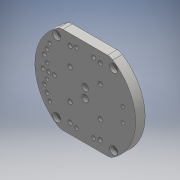
# Autodesk Inventor part: Modular Chassis
Saved by Autodesk Inventor 2016 (Build 200138000, 138)
## iProperties
Created: 2017-03-04
Part Number: Modular Chassis
Material: Generic
Document SubType Name: Modeling
Designer: Billy
Density: 1 g/cm^3
Appearance: Default
Author: Billy
Autodesk Inventor part; units mm, degrees
ref_plane "YZ Plane" through (0, 0, 0) normal (1, 0, 0) x (0, 1, 0)
ref_plane "XZ Plane" through (0, 0, 0) normal (0, 1, 0) x (-1, 0, 0)
ref_plane "XY Plane" through (0, 0, 0) normal (0, 0, 1) x (1, 0, 0)
sketch "Sketch1" plane through (0, 0, 0) normal (0, 1, 0) x (-1, 0, 0)
  circle A0 centre (15.9, 35) radius 2.25
  circle A1 centre (-15.9, 35) radius 2.25
  circle A2 centre (15.9, 16) radius 2.25
  circle A3 centre (-15.9, 16) radius 2.25
  circle A4 centre (0, 0) radius 50.311529
  circle A5 centre (15.9, -35) radius 2.25
  circle A6 centre (-15.9, -35) radius 2.25
  circle A7 centre (15.9, -16) radius 2.25
  circle A8 centre (-15.9, -16) radius 2.25
  circle A9 centre (9, 36.699372) radius 2
  circle A10 centre (-9, 36.699372) radius 2
  circle A11 centre (9, -36.699372) radius 2
  circle A12 centre (-9, -36.699372) radius 2
  circle A13 centre (39.811529, 7.366) radius 1.75
  circle A14 centre (39.811529, -7.366) radius 1.75
  circle A15 centre (-39.811529, 7.366) radius 1.75
  circle A16 centre (-39.811529, -7.366) radius 1.75
  circle A17 centre (27.855765, 21.183) radius 1.5
  circle A18 centre (30.740586, 14.805085) radius 1.5
  circle A19 centre (24.970943, 27.560915) radius 1.5
  circle A20 centre (27.855765, -21.183) radius 1.5
  circle A21 centre (30.740586, -14.805085) radius 1.5
  circle A22 centre (24.970943, -27.560915) radius 1.5
  circle A23 centre (0, 32.311529) radius 2
  circle A24 centre (0, 38.311529) radius 2
  circle A25 centre (0, 44.311529) radius 2
  circle A26 centre (-32.311529, 0) radius 2
  circle A27 centre (-38.311529, 0) radius 2
  circle A28 centre (-44.311529, 0) radius 2
  circle A29 centre (0, -32.311529) radius 2
  circle A30 centre (0, -38.311529) radius 2
  circle A31 centre (0, -44.311529) radius 2
  circle A32 centre (32.311529, 0) radius 2
  circle A33 centre (38.311529, 0) radius 2
  circle A34 centre (44.311529, 0) radius 2
  circle A35 centre (0, 5) radius 2.5
  circle A36 centre (0, -5) radius 2.5
  circle A37 centre (24.105765, 8) radius 2
  circle A38 centre (24.105765, -8) radius 2
  circle A39 centre (-24.105765, 8) radius 2
  circle A40 centre (-24.105765, -8) radius 2
  circle A41 centre (-27.855765, -21.183) radius 2
  circle A42 centre (27.885979, -37.390623) radius 2
  line L0 (0, 0) -> (2.5, 0)
  circle A43 centre (27.885979, 37.390623) radius 2
  circle A44 centre (44.311529, -14.732) radius 2
  circle A45 centre (44.311529, 14.732) radius 2
  line L1 (-27.855765, -21.183) -> (-36.920676, -29.026812)
  circle A46 centre (-21.877882, -28.0915) radius 2
  circle A47 centre (-33.833647, -14.2745) radius 2
  circle A48 centre (-27.927504, -33.3262) radius 2
  circle A49 centre (-33.905386, -26.4177) radius 2
  circle A50 centre (-39.883268, -19.5092) radius 2
  circle A51 centre (-27.855765, 21.183) radius 2
  circle A52 centre (-21.877882, 28.0915) radius 2
  circle A53 centre (-33.833647, 14.2745) radius 2
  circle A54 centre (-27.927504, 33.3262) radius 2
  circle A55 centre (-33.905386, 26.4177) radius 2
  circle A56 centre (-39.883268, 19.5092) radius 2
  circle A57 centre (36.098754, -26.061311) radius 2
  circle A58 centre (36.098754, 26.061311) radius 2
  point P0 (-36.920676, 29.026812)
  dimension "d47" = 360
  dimension "d64" = 8
  dimension "d69" = 4
  dimension "d70" = 4
  constraints: 59 centre point, 9 symmetric about line, 4 end point, 1 horizontal, 40 other
  measures "d64" distance of A46.centre A48.centre
  measures "d69" diameter of A57
  measures "d70" diameter of A58
extrude "Extrusion1" add sketch "Sketch1" along normal blind 10
sketch "Sketch2" plane through (0, 10, 0) normal (0, 1, 0) x (1, 0, 0)
  circle A0 centre (0, 5) radius 2.5
  circle A1 centre (0, -5) radius 2.5
  circle A2 centre (15.9, 16) radius 2.25
  circle A3 centre (-15.9, 16) radius 2.25
  circle A4 centre (15.9, 35) radius 2.25
  circle A5 centre (-15.9, 35) radius 2.25
  circle A6 centre (15.9, -16) radius 2.25
  circle A7 centre (-15.9, -16) radius 2.25
  circle A8 centre (15.9, -35) radius 2.25
  circle A9 centre (-36.098754, -26.061311) radius 2
  circle A10 centre (-36.098754, 26.061311) radius 2
  circle A11 centre (27.927504, -33.3262) radius 2
  circle A12 centre (39.883268, -19.5092) radius 2
  circle A13 centre (33.833647, -14.2745) radius 2
  circle A14 centre (27.855765, -21.183) radius 2
  circle A15 centre (33.905386, -26.4177) radius 2
  circle A16 centre (21.877882, -28.0915) radius 2
  circle A17 centre (39.883268, 19.5092) radius 2
  circle A18 centre (33.905386, 26.4177) radius 2
  circle A19 centre (27.927504, 33.3262) radius 2
  circle A20 centre (33.833647, 14.2745) radius 2
  circle A21 centre (21.877882, 28.0915) radius 2
  circle A22 centre (-44.311529, -14.732) radius 2
  circle A23 centre (-44.311529, 14.732) radius 2
  circle A24 centre (-27.885979, -37.390623) radius 2
  circle A25 centre (-27.885979, 37.390623) radius 2
  circle A26 centre (27.855765, 21.183) radius 2
  circle A27 centre (24.105765, 8) radius 2
  circle A28 centre (24.105765, -8) radius 2
  circle A29 centre (-24.105765, 8) radius 2
  circle A30 centre (-24.105765, -8) radius 2
  circle A31 centre (-44.311529, 0) radius 2
  circle A32 centre (-38.311529, 0) radius 2
  circle A33 centre (-32.311529, 0) radius 2
  circle A34 centre (0, 44.311529) radius 2
  circle A35 centre (0, 38.311529) radius 2
  circle A36 centre (0, 32.311529) radius 2
  circle A37 centre (44.311529, 0) radius 2
  circle A38 centre (38.311529, 0) radius 2
  circle A39 centre (32.311529, 0) radius 2
  circle A40 centre (0, -44.311529) radius 2
  circle A41 centre (0, -38.311529) radius 2
  circle A42 centre (0, -32.311529) radius 2
  circle A43 centre (-9, 36.699372) radius 2
  circle A44 centre (9, 36.699372) radius 2
  circle A45 centre (9, -36.699372) radius 2
  circle A46 centre (39.811529, 7.366) radius 1.75
  circle A47 centre (39.811529, -7.366) radius 1.75
  circle A48 centre (-39.811529, 7.366) radius 1.75
  circle A49 centre (-39.811529, -7.366) radius 1.75
  circle A50 centre (-30.740586, 14.805085) radius 1.5
  circle A51 centre (-27.855765, 21.183) radius 1.5
  circle A52 centre (-24.970943, 27.560915) radius 1.5
  circle A53 centre (-24.970943, -27.560915) radius 1.5
  circle A54 centre (-30.740586, -14.805085) radius 1.5
  circle A55 centre (-27.855765, -21.183) radius 1.5
  circle A56 centre (0, 0) radius 50.311529
  circle A57 centre (44.311529, 0) radius 2
  circle A58 centre (38.311529, 0) radius 2
  circle A59 centre (32.311529, 0) radius 2
  circle A60 centre (39.811529, 7.366) radius 1.75
  circle A61 centre (39.811529, -7.366) radius 1.75
  circle A62 centre (-15.9, -16) radius 5
  arc A63 (-14.704301, -30.145074) -> (-17.095699, -39.854926) centre (-15.9, -35) ccw
  arc A64 (-10.195699, -41.554298) -> (-7.804301, -31.844446) centre (-9, -36.699372) ccw
  line L0 (-10.195699, -41.554298) -> (-17.095699, -39.854926)
  circle A65 centre (-15.9, -35) radius 2.25
  circle A66 centre (-9, -36.699372) radius 2
  line L1 (-7.804301, -31.844446) -> (-14.704301, -30.145074)
  line L2 (0, 0) -> (0, -5)
  line L3 (0, 0) -> (-3.620732, 0)
  circle A67 centre (15.9, -16) radius 5
  arc A68 (17.095699, -39.854926) -> (14.704301, -30.145074) centre (15.9, -35) ccw
  arc A69 (7.804301, -31.844446) -> (10.195699, -41.554298) centre (9, -36.699372) ccw
  line L4 (10.195699, -41.554298) -> (17.095699, -39.854926)
  line L5 (7.804301, -31.844446) -> (14.704301, -30.145074)
  circle A70 centre (-15.9, 16) radius 5
  arc A71 (-17.095699, 39.854926) -> (-14.704301, 30.145074) centre (-15.9, 35) ccw
  arc A72 (-7.804301, 31.844446) -> (-10.195699, 41.554298) centre (-9, 36.699372) ccw
  line L6 (-10.195699, 41.554298) -> (-17.095699, 39.854926)
  line L7 (-7.804301, 31.844446) -> (-14.704301, 30.145074)
  arc A73 (14.704301, 30.145074) -> (17.095699, 39.854926) centre (15.9, 35) ccw
  line L8 (7.804301, 31.844446) -> (14.704301, 30.145074)
  arc A74 (10.195699, 41.554298) -> (7.804301, 31.844446) centre (9, 36.699372) ccw
  line L9 (10.195699, 41.554298) -> (17.095699, 39.854926)
  circle A75 centre (15.9, 16) radius 5
  circle A76 centre (-39.811529, 7.366) radius 4.25
  circle A77 centre (-39.811529, -7.366) radius 4.25
  circle A78 centre (39.811529, 7.366) radius 4.25
  circle A79 centre (39.811529, -7.366) radius 4.25
  dimension "d85" = 8.5
  dimension "d86" = 8.5
  dimension "d87" = 8.5
  dimension "d88" = 8.5
  constraints: 141 centre point, 21 symmetric about line, 20 end point, 16 point on circle, 5 coincident, 1 horizontal, 1 vertical, 9 other
  measures "d85" diameter of A76
  measures "d86" diameter of A77
  measures "d87" diameter of A78
  measures "d88" diameter of A79
extrude "Extrusion2" cut sketch "Sketch2" against normal blind 4 contours A62 | L1 A64 L0 A63 | A67 | L4 A69 L5 A68 | A70 | L6 A72 L7 A71 | L8 A74 L9 A73 | A75 | A76 | A77 | A78 | A79
sketch "Sketch3" plane through (0, 0, 0) normal (0, -1, 0) x (1, 0, 0)
  circle A0 centre (0, -5) radius 2.5
  circle A1 centre (0, 5) radius 2.5
  circle A2 centre (15.9, -16) radius 2.25
  circle A3 centre (-15.9, -16) radius 2.25
  circle A4 centre (15.9, -35) radius 2.25
  circle A5 centre (-15.9, -35) radius 2.25
  circle A6 centre (15.9, 16) radius 2.25
  circle A7 centre (-15.9, 16) radius 2.25
  circle A8 centre (15.9, 35) radius 2.25
  circle A9 centre (-15.9, 35) radius 2.25
  circle A10 centre (-36.098754, 26.061311) radius 2
  circle A11 centre (-36.098754, -26.061311) radius 2
  circle A12 centre (27.927504, 33.3262) radius 2
  circle A13 centre (39.883268, 19.5092) radius 2
  circle A14 centre (33.833647, 14.2745) radius 2
  circle A15 centre (27.855765, 21.183) radius 2
  circle A16 centre (33.905386, 26.4177) radius 2
  circle A17 centre (21.877882, 28.0915) radius 2
  circle A18 centre (39.883268, -19.5092) radius 2
  circle A19 centre (33.905386, -26.4177) radius 2
  circle A20 centre (27.927504, -33.3262) radius 2
  circle A21 centre (33.833647, -14.2745) radius 2
  circle A22 centre (21.877882, -28.0915) radius 2
  circle A23 centre (-44.311529, 14.732) radius 2
  circle A24 centre (-44.311529, -14.732) radius 2
  circle A25 centre (-27.885979, 37.390623) radius 2
  circle A26 centre (-27.885979, -37.390623) radius 2
  circle A27 centre (27.855765, -21.183) radius 2
  circle A28 centre (24.105765, -8) radius 2
  circle A29 centre (24.105765, 8) radius 2
  circle A30 centre (-24.105765, -8) radius 2
  circle A31 centre (-24.105765, 8) radius 2
  circle A32 centre (-44.311529, 0) radius 2
  circle A33 centre (-38.311529, 0) radius 2
  circle A34 centre (-32.311529, 0) radius 2
  circle A35 centre (0, -44.311529) radius 2
  circle A36 centre (0, -38.311529) radius 2
  circle A37 centre (0, -32.311529) radius 2
  circle A38 centre (44.311529, 0) radius 2
  circle A39 centre (38.311529, 0) radius 2
  circle A40 centre (32.311529, 0) radius 2
  circle A41 centre (0, 44.311529) radius 2
  circle A42 centre (0, 38.311529) radius 2
  circle A43 centre (0, 32.311529) radius 2
  circle A44 centre (-9, -36.699372) radius 2
  circle A45 centre (9, -36.699372) radius 2
  circle A46 centre (9, 36.699372) radius 2
  circle A47 centre (-9, 36.699372) radius 2
  circle A48 centre (39.811529, -7.366) radius 1.75
  circle A49 centre (39.811529, 7.366) radius 1.75
  circle A50 centre (-39.811529, -7.366) radius 1.75
  circle A51 centre (-39.811529, 7.366) radius 1.75
  circle A52 centre (-30.740586, -14.805085) radius 1.5
  circle A53 centre (-27.855765, -21.183) radius 1.5
  circle A54 centre (-24.970943, -27.560915) radius 1.5
  circle A55 centre (-24.970943, 27.560915) radius 1.5
  circle A56 centre (-30.740586, 14.805085) radius 1.5
  circle A57 centre (-27.855765, 21.183) radius 1.5
  circle A58 centre (0, 0) radius 50.311529
  arc A59 (-34.612892, 16.556584) -> (-26.868281, 13.053586) centre (-30.740586, 14.805085) ccw
  arc A60 (-21.098637, 25.809416) -> (-28.843249, 29.312414) centre (-24.970943, 27.560915) ccw
  line L0 (-28.843249, 29.312414) -> (-34.612892, 16.556584)
  line L1 (-21.098637, 25.809416) -> (-26.868281, 13.053586)
  line L2 (0, 0) -> (-2, 0)
  arc A61 (-26.868281, -13.053586) -> (-34.612892, -16.556584) centre (-30.740586, -14.805085) ccw
  arc A62 (-28.843249, -29.312414) -> (-21.098637, -25.809416) centre (-24.970943, -27.560915) ccw
  line L3 (-28.843249, -29.312414) -> (-34.612892, -16.556584)
  line L4 (-21.098637, -25.809416) -> (-26.868281, -13.053586)
  arc A63 (-32.311529, -4.25) -> (-32.311529, 4.25) centre (-32.311529, 0) ccw
  line L5 (-44.311529, -4.25) -> (-32.311529, -4.25)
  line L6 (-44.311529, 4.25) -> (-32.311529, 4.25)
  arc A64 (-44.311529, 4.25) -> (-44.311529, -4.25) centre (-44.311529, 0) ccw
  line L7 (0, 0) -> (0, 0.900681)
  arc A65 (32.311529, 4.25) -> (32.311529, -4.25) centre (32.311529, 0) ccw
  line L8 (44.311529, -4.25) -> (32.311529, -4.25)
  line L9 (44.311529, 4.25) -> (32.311529, 4.25)
  arc A66 (44.311529, -4.25) -> (44.311529, 4.25) centre (44.311529, 0) ccw
  arc A67 (-4.25, -44.311529) -> (4.25, -44.311529) centre (0, -44.311529) ccw
  arc A68 (4.25, -32.311529) -> (-4.25, -32.311529) centre (0, -32.311529) ccw
  line L10 (-4.25, -44.311529) -> (-4.25, -32.311529)
  line L11 (4.25, -32.311529) -> (4.25, -44.311529)
  arc A69 (4.25, 44.311529) -> (-4.25, 44.311529) centre (0, 44.311529) ccw
  arc A70 (-4.25, 32.311529) -> (4.25, 32.311529) centre (0, 32.311529) ccw
  line L12 (-4.25, 44.311529) -> (-4.25, 32.311529)
  line L13 (4.25, 32.311529) -> (4.25, 44.311529)
  constraints: 129 centre point, 28 end point, 24 point on circle, 18 symmetric about line, 6 coincident, 3 tangent, 2 horizontal, 1 vertical, 6 other
extrude "Extrusion3" cut sketch "Sketch3" against normal blind 4 contours L0 A60 L1 A59 | L4 A62 L3 A61 | L5 A64 L6 A63 | L9 A66 L8 A65 | L10 A68 L11 A67 | L13 A70 L12 A69
sketch "Sketch4" plane through (0, 10, 0) normal (0, 1, 0) x (1, 0, 0)
  circle A0 centre (-27.885979, -37.390623) radius 2
  circle A1 centre (-27.885979, 37.390623) radius 2
  point P0 (0, 0)
extrude "Extrusion4" add sketch "Sketch4" against normal blind 10
sketch "Sketch5" plane through (0, 10, 0) normal (0, 1, 0) x (1, 0, 0)
  line L0 (0, 0) -> (-30, 0)
  line L1 (-30, 37.5) -> (0, 37.5)
  line L2 (0, 37.5) -> (0, 0)
  line L3 (30, -37.5) -> (-30, -37.5)
  circle A0 centre (-30, -37.5) radius 2
  circle A1 centre (-30, 37.5) radius 2
  circle A2 centre (30, -37.5) radius 2
  circle A3 centre (30, 37.5) radius 2
  dimension "d104" = 30
  dimension "d105" = 37.5
  dimension "d106" = 60
  dimension "d108" = 4
  dimension "d109" = 4
  dimension "d110" = 4
  dimension "d111" = 4
  constraints: 8 end point, 4 centre point, 3 coincident, 1 horizontal, 1 parallel
  measures "d104" distance of L1.start L1.end
  measures "d105" distance of L0.end L1.start
  measures "d106" distance of L3.start L3.end
  measures "d108" diameter of A0
  measures "d109" diameter of A1
  measures "d110" diameter of A2
  measures "d111" diameter of A3
extrude "Extrusion5" cut sketch "Sketch5" against normal blind 10
sketch "Sketch6" plane through (0, 10, 0) normal (0, 1, 0) x (1, 0, 0)
  circle A0 centre (0, 0) radius 50.311529
  circle A1 centre (27.855765, 21.183) radius 2
  circle A2 centre (30, -37.5) radius 2
  circle A3 centre (-30, -37.5) radius 2
  circle A4 centre (-30, 37.5) radius 2
  circle A5 centre (30, 37.5) radius 2
  line L0 (-17.095699, 39.854926) -> (-10.195699, 41.554298)
  arc A6 (-7.804301, 31.844446) -> (-10.195699, 41.554298) centre (-9, 36.699372) ccw
  line L1 (-7.804301, 31.844446) -> (-14.704301, 30.145074)
  arc A7 (-17.095699, 39.854926) -> (-14.704301, 30.145074) centre (-15.9, 35) ccw
  line L2 (-14.704301, -30.145074) -> (-7.804301, -31.844446)
  arc A8 (-10.195699, -41.554298) -> (-7.804301, -31.844446) centre (-9, -36.699372) ccw
  line L3 (-10.195699, -41.554298) -> (-17.095699, -39.854926)
  arc A9 (-14.704301, -30.145074) -> (-17.095699, -39.854926) centre (-15.9, -35) ccw
  circle A10 centre (-15.9, 16) radius 5
  circle A11 centre (-15.9, -16) radius 5
  circle A12 centre (39.811529, 7.366) radius 4.25
  circle A13 centre (-39.811529, 7.366) radius 4.25
  circle A14 centre (-39.811529, -7.366) radius 4.25
  circle A15 centre (39.811529, -7.366) radius 4.25
  circle A16 centre (15.9, -16) radius 5
  circle A17 centre (15.9, 16) radius 5
  arc A18 (7.804301, -31.844446) -> (10.195699, -41.554298) centre (9, -36.699372) ccw
  line L4 (7.804301, -31.844446) -> (14.704301, -30.145074)
  arc A19 (17.095699, -39.854926) -> (14.704301, -30.145074) centre (15.9, -35) ccw
  line L5 (17.095699, -39.854926) -> (10.195699, -41.554298)
  arc A20 (14.704301, 30.145074) -> (17.095699, 39.854926) centre (15.9, 35) ccw
  line L6 (14.704301, 30.145074) -> (7.804301, 31.844446)
  arc A21 (10.195699, 41.554298) -> (7.804301, 31.844446) centre (9, 36.699372) ccw
  line L7 (10.195699, 41.554298) -> (17.095699, 39.854926)
  circle A22 centre (0, 5) radius 2.5
  circle A23 centre (0, -5) radius 2.5
  circle A24 centre (-36.098754, -26.061311) radius 2
  circle A25 centre (-36.098754, 26.061311) radius 2
  circle A26 centre (27.927504, -33.3262) radius 2
  circle A27 centre (39.883268, -19.5092) radius 2
  circle A28 centre (33.833647, -14.2745) radius 2
  circle A29 centre (27.855765, -21.183) radius 2
  circle A30 centre (33.905386, -26.4177) radius 2
  circle A31 centre (21.877882, -28.0915) radius 2
  circle A32 centre (39.883268, 19.5092) radius 2
  circle A33 centre (33.905386, 26.4177) radius 2
  circle A34 centre (27.927504, 33.3262) radius 2
  circle A35 centre (33.833647, 14.2745) radius 2
  circle A36 centre (21.877882, 28.0915) radius 2
  circle A37 centre (-44.311529, -14.732) radius 2
  circle A38 centre (-44.311529, 14.732) radius 2
  circle A39 centre (27.855765, 21.183) radius 2
  circle A40 centre (24.105765, 8) radius 2
  circle A41 centre (24.105765, -8) radius 2
  circle A42 centre (-24.105765, 8) radius 2
  circle A43 centre (-24.105765, -8) radius 2
  circle A44 centre (-44.311529, 0) radius 2
  circle A45 centre (-38.311529, 0) radius 2
  circle A46 centre (-32.311529, 0) radius 2
  circle A47 centre (0, 44.311529) radius 2
  circle A48 centre (0, 38.311529) radius 2
  circle A49 centre (0, 32.311529) radius 2
  circle A50 centre (44.311529, 0) radius 2
  circle A51 centre (38.311529, 0) radius 2
  circle A52 centre (32.311529, 0) radius 2
  circle A53 centre (0, -44.311529) radius 2
  circle A54 centre (0, -38.311529) radius 2
  circle A55 centre (0, -32.311529) radius 2
  circle A56 centre (-30.740586, 14.805085) radius 1.5
  circle A57 centre (-27.855765, 21.183) radius 1.5
  circle A58 centre (-24.970943, 27.560915) radius 1.5
  circle A59 centre (-24.970943, -27.560915) radius 1.5
  circle A60 centre (-30.740586, -14.805085) radius 1.5
  circle A61 centre (-27.855765, -21.183) radius 1.5
  circle A62 centre (0, 0) radius 50.311529
  circle A63 centre (0, 0) radius 53
  dimension "d115" = 106
  constraints: 1 centre point, 1 coincident
  measures "d115" diameter of A63
extrude "Extrusion6" add sketch "Sketch6" against normal blind 10 contours A1 | A26 | A27 | A28 | A29 | A30 | A31 | A32 | A33 | A34 | A35 | A36 | A63
sketch "Sketch8" plane through (0, 0, 0) normal (0, -1, 0) x (1, 0, 0)
  circle A0 centre (30, -37.5) radius 2 projected
  circle A1 centre (30, -37.5) radius 4.25
  circle A2 centre (30, 37.5) radius 2 projected
  circle A3 centre (30, 37.5) radius 4.25
  circle A4 centre (-30, 37.5) radius 2 projected
  circle A5 centre (-30, 37.5) radius 4.25
  circle A6 centre (-30, -37.5) radius 2 projected
  circle A7 centre (-30, -37.5) radius 4.25
  point P0 (0, 0)
  dimension "d118" = 8.5
  dimension "d119" = 8.5
  dimension "d120" = 8.5
  dimension "d121" = 8.5
  constraints: 4 centre point, 4 coincident
  measures "d118" diameter of A1
  measures "d119" diameter of A3
  measures "d120" diameter of A5
  measures "d121" diameter of A7
extrude "Extrusion7" cut sketch "Sketch8" against normal blind 4
move faces "Move2" translate (0, -4, 0) faces at (-24.8315, 4, -19.782972) (-30.88003, 4, 22.583028)
sketch "Sketch11" plane through (0, 0, 0) normal (0, -1, 0) x (1, 0, 0)
  line L0 (32.311529, 4.25) -> (44.311529, 4.25)
  arc A0 (32.311529, 4.25) -> (32.311529, -4.25) centre (32.311529, 0) ccw
  line L1 (44.311529, -4.25) -> (32.311529, -4.25)
  arc A1 (44.311529, -4.25) -> (44.311529, 4.25) centre (44.311529, 0) ccw
  circle A2 centre (32.311529, 0) radius 2
  circle A3 centre (38.311529, 0) radius 2
  circle A4 centre (44.311529, 0) radius 2
  line L2 (32.311529, 4.25) -> (44.311529, 4.25)
  arc A5 (32.311529, 4.25) -> (32.311529, -4.25) centre (32.311529, 0) ccw
  line L3 (44.311529, -4.25) -> (32.311529, -4.25)
  arc A6 (44.311529, -4.25) -> (44.311529, 4.25) centre (44.311529, 0) ccw
  circle A7 centre (-36.098754, 26.061311) radius 2
  circle A8 centre (-44.311529, 14.732) radius 2
  circle A9 centre (-44.311529, -14.732) radius 2
  circle A10 centre (-36.098754, -26.061311) radius 2
  point P0 (0, 0)
extrude "Extrusion8" add sketch "Sketch11" against normal blind 10 contours L0 A1 L1 A0 | A2 | A3 | A4 | A7 | A8 | A9 | A10
sketch "Sketch12" plane through (0, 0, 0) normal (0, -1, 0) x (1, 0, 0)
  circle A0 centre (-30.740586, -14.805085) radius 1.5
  circle A1 centre (-27.855765, -21.183) radius 1.5
  circle A2 centre (-24.970943, -27.560915) radius 1.5
  circle A3 centre (-30.740586, 14.805085) radius 1.5
  circle A4 centre (-27.855765, 21.183) radius 1.5
  circle A5 centre (-24.970943, 27.560915) radius 1.5
  point P0 (0, 0)
extrude "Extrusion9" add sketch "Sketch12" against normal blind 10
sketch "Sketch13" plane through (0, 0, 0) normal (0, -1, 0) x (1, 0, 0)
  line L0 (0, 0) -> (-180, 0)
  line L1 (-180, 0) -> (-180, 80)
  line L2 (-180, 80) -> (0, 80)
  line L3 (0, 80) -> (0, 0)
  circle A0 centre (-40, 20) radius 2
  circle A1 centre (-42.757435, 13.565985) radius 2
  circle A2 centre (-37.242565, 26.434015) radius 2
  circle A3 centre (-40, -20) radius 2
  circle A4 centre (-42.757435, -13.565985) radius 2
  circle A5 centre (-37.242565, -26.434015) radius 2
  dimension "d133" = 180
  dimension "d134" = 80
  constraints: 8 end point, 6 centre point, 3 symmetric about line, 2 parallel, 1 horizontal, 1 perpendicular, 3 other
  measures "d133" distance of L1.end L2.end
  measures "d134" distance of L0.end L1.end
extrude "Extrusion10" cut sketch "Sketch13" against normal blind 10 contours A0 | A1 | A2 | A3 | A4 | A5
sketch "Sketch15" plane through (0, 10, 0) normal (0, 1, 0) x (1, 0, 0)
  line L0 (-33.336199, -24.759858) -> (-38.096595, -13.652267)
  arc A0 (-41.148931, -28.108172) -> (-33.336199, -24.759858) centre (-37.242565, -26.434015) ccw
  line L1 (-41.148931, -28.108172) -> (-46.663801, -15.240142)
  arc A1 (-36.046217, -9.33702) -> (-43.717896, -5.691843) centre (-39.811529, -7.366) ccw
  line L2 (-43.717896, -5.691843) -> (-46.663801, -11.891828)
  line L3 (-35.905163, -9.040157) -> (-38.096595, -13.652267)
  arc A2 (-46.522748, -11.594965) -> (-46.663801, -15.240142) centre (-42.757435, -13.565985) ccw
  line L4 (0, 0) -> (-4.988215, 0)
  line L5 (-33.336199, 24.759858) -> (-38.096595, 13.652267)
  arc A3 (-33.336199, 24.759858) -> (-41.148931, 28.108172) centre (-37.242565, 26.434015) ccw
  line L6 (-41.148931, 28.108172) -> (-46.663801, 15.240142)
  arc A4 (-43.717896, 5.691843) -> (-36.046217, 9.33702) centre (-39.811529, 7.366) ccw
  line L7 (-43.717896, 5.691843) -> (-46.663801, 11.891828)
  line L8 (-35.905163, 9.040157) -> (-38.096595, 13.652267)
  arc A5 (-46.663801, 15.240142) -> (-46.522748, 11.594965) centre (-42.757435, 13.565985) ccw
  constraints: 18 end point, 12 point on circle, 12 symmetric about line, 6 centre point, 4 point on line, 1 horizontal, 3 other
extrude "Extrusion11" cut sketch "Sketch15" against normal blind 4
sketch "Sketch17" plane through (0, 10, 0) normal (0, 1, 0) x (1, 0, 0)
  arc A0 (-48.533913, 0.483709) -> (-48.533913, -0.483709) centre (-44.311529, 0) ccw
  arc A1 (-29.333535, -3.032169) -> (-29.333535, 3.032169) centre (-32.311529, 0) ccw
  line L0 (-36.302701, -9.876819) -> (-38.096595, -13.652267)
  circle A2 centre (-42.757435, -13.565985) radius 2
  arc A3 (-46.979819, -14.049693) -> (-46.663801, -15.240142) centre (-42.757435, -13.565985) ccw
  line L1 (-36.302701, -9.876819) -> (-29.333535, -3.032169)
  line L2 (-46.979819, -14.049693) -> (-48.533913, -0.483709)
  line L3 (-38.096595, -13.652267) -> (-33.336199, -24.759858)
  arc A4 (-41.148931, -28.108172) -> (-33.336199, -24.759858) centre (-37.242565, -26.434015) ccw
  line L4 (-41.148931, -28.108172) -> (-46.663801, -15.240142)
  line L5 (0, 0) -> (-2.144861, 0)
  arc A5 (-29.333535, -3.032169) -> (-29.333535, 3.032169) centre (-32.311529, 0) ccw
  line L6 (-36.302701, 9.876819) -> (-38.096595, 13.652267)
  circle A6 centre (-42.757435, 13.565985) radius 2
  arc A7 (-46.663801, 15.240142) -> (-46.979819, 14.049693) centre (-42.757435, 13.565985) ccw
  line L7 (-36.302701, 9.876819) -> (-29.333535, 3.032169)
  line L8 (-46.979819, 14.049693) -> (-48.533913, 0.483709)
  line L9 (-38.096595, 13.652267) -> (-33.336199, 24.759858)
  arc A8 (-33.336199, 24.759858) -> (-41.148931, 28.108172) centre (-37.242565, 26.434015) ccw
  line L10 (-41.148931, 28.108172) -> (-46.663801, 15.240142)
  constraints: 22 end point, 14 point on circle, 9 centre point, 1 horizontal
extrude "Extrusion13" cut sketch "Sketch17" against normal blind 4
sketch "Sketch18" plane through (0, 10, 0) normal (0, 1, 0) x (1, 0, 0)
  circle A0 centre (39.811529, -7.366) radius 1.75
  circle A1 centre (39.811529, -7.366) radius 4.25
  arc A2 (42.701693, 4.25) -> (36.921366, 4.25) centre (39.811529, 7.366) ccw
  circle A3 centre (39.811529, 7.366) radius 4.25
  point P0 (0, 0)
  constraints: 2 coincident, 1 centre point, 3 other
extrude "Extrusion14" cut sketch "Sketch18" against normal blind 4
sketch "Sketch19" plane through (0, 0, 0) normal (0, -1, 0) x (1, 0, 0)
  arc A0 (-32.311529, -4.25) -> (-32.311529, 4.25) centre (-32.311529, 0) ccw
  line L0 (-44.311529, 4.25) -> (-32.311529, 4.25)
  arc A1 (-44.311529, 4.25) -> (-44.311529, -4.25) centre (-44.311529, 0) ccw
  line L1 (-32.311529, -4.25) -> (-44.311529, -4.25)
  circle A2 centre (-44.311529, 0) radius 2
  circle A3 centre (-38.311529, 0) radius 2
  circle A4 centre (-32.311529, 0) radius 2
  point P0 (0, 0)
extrude "Extrusion15" add sketch "Sketch19" against normal blind 4
sketch "Sketch21" plane through (0, 0, 0) normal (0, -1, 0) x (1, 0, 0)
  line L0 (-4.25, -44.311529) -> (-4.25, -32.311529)
  arc A0 (4.25, -32.311529) -> (-4.25, -32.311529) centre (0, -32.311529) ccw
  line L1 (4.25, -32.311529) -> (4.25, -44.311529)
  arc A1 (-4.25, -44.311529) -> (4.25, -44.311529) centre (0, -44.311529) ccw
  arc A2 (-4.25, 32.311529) -> (4.25, 32.311529) centre (0, 32.311529) ccw
  line L2 (-4.25, 32.311529) -> (-4.25, 44.311529)
  arc A3 (4.25, 44.311529) -> (-4.25, 44.311529) centre (0, 44.311529) ccw
  line L3 (4.25, 44.311529) -> (4.25, 32.311529)
  point P0 (0, 0)
extrude "Extrusion16" add sketch "Sketch21" against normal blind 10
sketch "Sketch22" plane through (0, 10, 0) normal (0, 1, 0) x (1, 0, 0)
  line L0 (0, -46) -> (-26.324893, -46)
  line L1 (0, -46) -> (26.324893, -46)
  line L2 (0, 0) -> (-4.64363, 0)
  line L3 (0, 46) -> (-26.324893, 46)
  line L4 (0, 46) -> (26.324893, 46)
  arc A0 (-26.324893, -46) -> (26.324893, -46) centre (0, 0) ccw
  arc A1 (26.324893, 46) -> (-26.324893, 46) centre (0, 0) ccw
  constraints: 10 end point, 4 point on circle, 2 centre point, 2 point on line
extrude "Extrusion17" cut sketch "Sketch22" against normal blind 10
fillet "Fillet1" radius 10 4 edges at (26.3249, 5, 46) (-26.3249, 5, 46) (26.3249, 5, -46) (-26.3249, 5, -46)
sketch "Sketch23" plane through (0, 10, 0) normal (0, 1, 0) x (1, 0, 0)
  circle A0 centre (0, -5) radius 2.5 projected
  circle A1 centre (0, -5) radius 3.5
  circle A2 centre (0, 5) radius 2.5 projected
  circle A3 centre (0, 5) radius 3.5
  point P0 (0, 0)
  dimension "d163" = 7
  dimension "d164" = 7
  constraints: 2 centre point, 2 coincident
  measures "d163" diameter of A1
  measures "d164" diameter of A3
extrude "Extrusion18" cut sketch "Sketch23" against normal blind 10
sketch "Sketch24" plane through (0, 10, 0) normal (0, 1, 0) x (1, 0, 0)
  circle A0 centre (-24.105765, -8) radius 2
  circle A1 centre (-24.105765, 8) radius 2
  circle A2 centre (24.105765, 8) radius 2
  circle A3 centre (24.105765, -8) radius 2
  point P0 (0, 0)
extrude "Extrusion19" add sketch "Sketch24" against normal blind 10
sketch "Sketch25" plane through (0, 10, 0) normal (0, 1, 0) x (1, 0, 0)
  arc A0 (-4.25, 38.260621) -> (-10.195699, 41.554298) centre (-9, 36.699372) ccw
  circle A1 centre (-9, 36.699372) radius 5
  arc A2 (10.195699, 41.554298) -> (4.25, 38.260621) centre (9, 36.699372) ccw
  circle A3 centre (9, 36.699372) radius 5
  arc A4 (-4.25, -35.138122) -> (-7.804301, -31.844446) centre (-9, -36.699372) ccw
  circle A5 centre (-9, -36.699372) radius 5
  circle A6 centre (9, -36.699372) radius 2
  arc A7 (7.804301, -31.844446) -> (4.25, -35.138122) centre (9, -36.699372) ccw
  circle A8 centre (9, -36.699372) radius 5
  point P0 (0, 0)
  constraints: 4 coincident, 2 centre point, 6 other
extrude "Extrusion20" cut sketch "Sketch25" against normal blind 4
body "Solid1"
